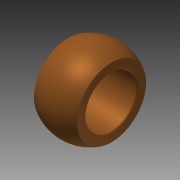
# Autodesk Inventor part: 1410P
Saved by Autodesk Inventor 2013 (Build 170138000, 138)
## iProperties
Category: Miscellaneous
Company: Autodesk Inc.
Created: 2012-12-03
Part Number: 1410P
Document SubType Name: Modeling
Designer: Autodesk Inc.
Density: 1 g/cm^3
Material: Generic
Author: Autodesk Inc.
Autodesk Inventor part; units mm, degrees
ref_plane "YZ Plane" through (0, 0, 0) normal (1, 0, 0) x (0, 1, 0)
ref_plane "XZ Plane" through (0, 0, 0) normal (0, 1, 0) x (-1, 0, 0)
ref_plane "XY Plane" through (0, 0, 0) normal (0, 0, 1) x (1, 0, 0)
sketch "Sketch1" plane through (0, 0, 0) normal (0, 0, 1) x (1, 0, 0)
  arc A0 (103.6702, 18.7694) -> (117.1276, 18.7694) centre (110.3989, 29.5404) ccw
  line L0 (103.6702, 40.3608) -> (103.6702, 29.5898)
  line L1 (117.1276, 40.3608) -> (117.1276, 29.5898)
  line L2 (95.2163, 29.5898) -> (125.5815, 29.5898)
  arc A1 (117.1276, 40.3608) -> (103.6702, 40.3608) centre (110.3989, 29.5898) ccw
  point P0 (0, 0)
  point P1 (110.3989, 16.8404)
  dimension "d44" = 21.6408
  dimension "d45" = 12.7
  dimension "d46" = 12.7
  constraints: 6 end point, 5 point on circle, 2 centre point, 2 point on line, 1 coincident, 1 midpoint, 1 parallel, 1 perpendicular, 1 vertical, 1 vertical alignment
  measures "d44" diameter of A0.start L2
  measures "d45" radius of A1
  measures "d46" radius of A0
revolve "Revolution1" add sketch "Sketch1" angle 360 about axis through (95.2163, 29.5898, 0) along (1, 0, 0)
sketch "Sketch2" plane through (117.1276, 29.5898, 0) normal (1, 0, 0) x (0, 0, -1)
  circle A0 centre (0, 0) radius 10.771 projected
  point P0 (0, -29.5898)
hole "Hole1" at (117.1276, 29.5898, 0) direction (-1, 0, 0) diameter 15.9258 depth 25.4 tip angle 118
chamfer "Chamfer1" distance 0.254 angle 45 2 edges at (117.1276, 29.5898, 7.9629) (103.6702, 29.5898, 7.9629)
equation "\"d45\" = d46"
body "Solid1"
